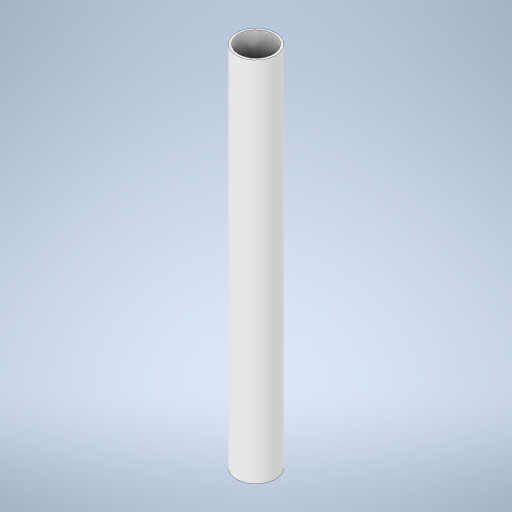
# Autodesk Inventor part: base
Saved by Autodesk Inventor 2024.3 (Build 283343000, 343)
## iProperties
Created: 2024-10-09
Part Number: base
Material: Generic
Document SubType Name: Modeling
Designer: pjcaa
Density: 1 g/cm^3
Appearance: Default(1)
Author: pjcaa
Autodesk Inventor part; units mm, degrees
ref_plane "YZ Plane" through (0, 0, 0) normal (1, 0, 0) x (0, 1, 0)
ref_plane "XZ Plane" through (0, 0, 0) normal (0, 1, 0) x (-1, 0, 0)
ref_plane "XY Plane" through (0, 0, 0) normal (0, 0, 1) x (1, 0, 0)
sketch "Sketch15" plane through (0, 0, 0) normal (0, 0, 1) x (1, 0, 0)
  circle A0 centre (0, 0) radius 10.7
  circle A1 centre (0, 0) radius 9.5
  dimension "d74" = 21.4
  dimension "d75" = 19
  constraints: 2 centre point, 2 coincident
  measures "d74" diameter of A0
  measures "d75" diameter of A1
extrude "Extrusion15" add sketch "Sketch15" along normal blind 200
body "Solid3"
